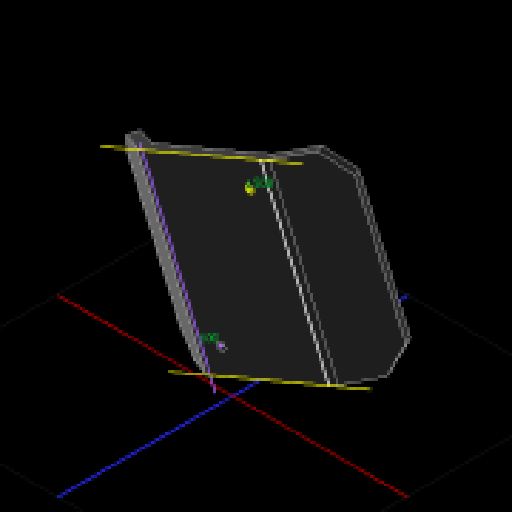
# Autodesk Inventor part: aligner
Saved by Autodesk Inventor 2025.2 (Build 292293000, 293)
## iProperties
Created: 2026-01-05
Part Number: aligner
Material: Acetal Resin, Black
Document SubType Name: Modeling
Designer: cloudy
Density: 1.425 g/cm^3
Appearance: Smooth - Black
Author: cloudy
Autodesk Inventor part; units mm, degrees
ref_plane "YZ Plane" through (0, 0, 0) normal (1, 0, 0) x (0, 1, 0)
ref_plane "XZ Plane" through (0, 0, 0) normal (0, 1, 0) x (-1, 0, 0)
ref_plane "XY Plane" through (0, 0, 0) normal (0, 0, 1) x (1, 0, 0)
sketch "Sketch1" plane through (0, 0, 0) normal (0, 0, 1) x (1, 0, 0)
  circle A0 centre (5.0561, -7.4217) radius 3.0353 construction
  circle A1 centre (21.615, 79.9226) radius 3.0353 construction
  line L0 (103.3314, 19.2847) -> (-36.9389, -40.2973)
  line L1 (-36.9389, -40.2973) -> (-76.6602, 53.2162)
  line L2 (-76.6602, 53.2162) -> (63.61, 112.7982)
  line L3 (63.61, 112.7982) -> (103.3314, 19.2847)
  line L4 (103.3314, 19.2847) -> (-76.6602, 53.2162) construction
  line L5 (-36.9389, -40.2973) -> (63.61, 112.7982) construction
  line L6 (33.1962, -10.5063) -> (-6.5251, 83.0072) construction
  line L7 (-55.6349, 168.7379) -> (0.8706, 192.7395) projected
  circle A2 centre (21.615, 79.9226) radius 2.1844
  circle A3 centre (5.0561, -7.4217) radius 2.1844
  circle A4 centre (26.6711, 72.5009) radius 2.1844 construction
  circle A5 centre (26.6711, 72.5009) radius 2.2479
  point P0 (0, 0)
  point P1 (13.3356, 36.2505)
  dimension "d0" = 101.6
  dimension "d1" = 152.4
  dimension "d5" = 49.3889
  dimension "d6" = 49.3889
  dimension "d7" = 13.8407
  dimension "d8" = 13.8407
  dimension "d22" = 4.3688
  dimension "d23" = 4.3688
  dimension "d25" = 4.4958
  constraints: 14 end point, 4 midpoint, 3 centre point, 3 coincident, 3 parallel, 1 perpendicular
  measures "d0" distance of L0.end L1.end
  measures "d1" distance of L1.end L2.end
  measures "d5" diameter of A0.centre L6
  measures "d6" diameter of A1.centre L6
  measures "d7" distance from line of L2 A1.centre
  measures "d8" distance from line of L0 A0.centre
  measures "d22" diameter of A2
  measures "d23" diameter of A3
  measures "d25" diameter of A5
extrude "Extrusion1" add sketch "Sketch1" along normal blind 6.35 contours L0 L1 L2 L3 | A2
chamfer "Chamfer1" distance 12.7 angle 45 4 edges at (103.3314, 19.2847, 3.175) (63.61, 112.7982, 3.175) (-76.6602, 53.2162, 3.175) (-36.9389, -40.2973, 3.175)
sketch "Sketch2" plane through (0, 0, 6.35) normal (0, 0, 1) x (1, 0, 0)
  line L0 (-25.2497, -35.3321) -> (91.6422, 14.3195) projected
  line L1 (66.0017, 3.4283) -> (26.2804, 96.9419)
  line L2 (51.9209, 107.833) -> (-64.971, 58.1814) projected
  line L3 (-47.1373, 78.4883) -> (-3.2385, -24.8602)
  circle A0 centre (16.5589, 87.3442) radius 2.1844 projected
  point P0 (0, 0)
  point P1 (0, 0)
  dimension "d14" = 12.7
  dimension "d24" = 12.7
  constraints: 4 end point, 2 perpendicular, 2 point on line
  measures "d14" distance from line of L3 point (0, 0)
  measures "d24" distance from line of L1 A0.centre
bend part "Bend Part1" radius 8.89 angle 30 line through (66.0017, 3.4283, 6.35) along (-0.3909577, 0.9204086, 0) centre toward (0, 0, -1) moving side (0.9204086, 0.3909577, 0) both sides no
bend part "Bend Part2" radius 8.89 angle 30 line through (-47.1373, 78.4883, 6.35) along (0.3909577, -0.9204086, 0) centre toward (0, 0, -1) moving side (-0.9204086, -0.3909577, 0) both sides no
ref_plane "Work Plane1" through (-22.6953, 20.9458, 0) normal (0.3909577, -0.9204086, 0) x (0.9204086, 0.3909577, 0)
sketch "Sketch3" plane through (-22.6953, 20.9458, 0) normal (0.3909577, -0.9204086, 0) x (0.9204086, 0.3909577, 0)
  line L0 (-18.3295, -10.1896) -> (-1.27, -0.3403) projected
  line L1 (0, 0) -> (74.7889, 0) projected
  line L2 (76.0589, -0.3403) -> (96.1532, -11.9417) projected
  line L3 (96.1532, -11.9417) -> (107.1517, -18.2917) projected
  line L4 (-29.3281, -16.5396) -> (-18.3295, -10.1896) projected
  line L5 (-21.7083, -15.875) -> (96.1532, -15.875)
  point P0 (12.7, 0)
  dimension "d33" = 15.875
  constraints: 2 end point, 1 horizontal
  measures "d33" distance between parallel lines of L1 L5
extrude "Rib1" add sketch "Sketch3" along normal mid plane 5.08 rib yes fills toward (37.2225, -15.825) open curves L5
fillet "Fillet1" radius 3.175 12 edges at (72.0753, 61.2011, -15.875) (45.7531, 52.78, -0.0865) (10.7299, 37.9033, 0) (-24.2934, 23.0266, -0.0865) (-37.2399, 17.5274, -8.1076) (58.6996, 58.2792, -8.1076) (47.7392, 48.1043, -0.0865) (60.6857, 53.6035, -8.1076) (-22.3073, 18.3509, -0.0865) (-35.2538, 12.8517, -8.1076) (12.7159, 33.2276, 0) (-48.6295, 9.9298, -15.875)
equation "\"d5\" = d6"
equation "\"d7\" = d8"
body "Solid1"
